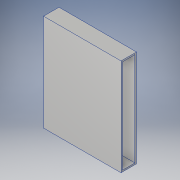
# Autodesk Inventor part: Motor Mount
Saved by Autodesk Inventor 2019.4 (Build 234330000, 330)
## iProperties
Created: 2019-10-20
Part Number: Motor Mount
Material: Aluminum 6061
Document SubType Name: Modeling
Designer: admin
Density: 2.7 g/cm^3
Appearance: Aluminum - Flat
Author: admin
Autodesk Inventor part; units mm, degrees
ref_plane "YZ Plane" through (0, 0, 0) normal (1, 0, 0) x (0, 1, 0)
ref_plane "XZ Plane" through (0, 0, 0) normal (0, 1, 0) x (-1, 0, 0)
ref_plane "XY Plane" through (0, 0, 0) normal (0, 0, 1) x (1, 0, 0)
sketch "Sketch1" plane through (0, 0, 0) normal (1, 0, 0) x (0, 1, 0)
  line L0 (-62.5, 10) -> (62.5, 10)
  line L1 (62.5, 10) -> (62.5, -10)
  line L2 (62.5, -10) -> (-62.5, -10)
  line L3 (-62.5, -10) -> (-62.5, 10)
  line L4 (-62.5, 10) -> (62.5, -10) construction
  line L5 (62.5, 10) -> (-62.5, -10) construction
  line L6 (60.5, -8) -> (60.5, 8)
  line L7 (60.5, 8) -> (-60.5, 8)
  line L8 (-60.5, 8) -> (-60.5, -8)
  line L9 (-60.5, -8) -> (60.5, -8)
  point P0 (0, 0)
  dimension "d0" = 125
  dimension "d1" = 20
  dimension "d2" = 2
  constraints: 20 end point, 4 parallel, 2 midpoint, 2 perpendicular, 1 horizontal, 3 other
  measures "d0" distance of L1.end L2.end
  measures "d1" distance of L0.end L1.end
  measures "d2" distance between parallel lines of L1 L6
extrude "Extrusion1" add sketch "Sketch1" along normal blind 100
body "Solid1"
